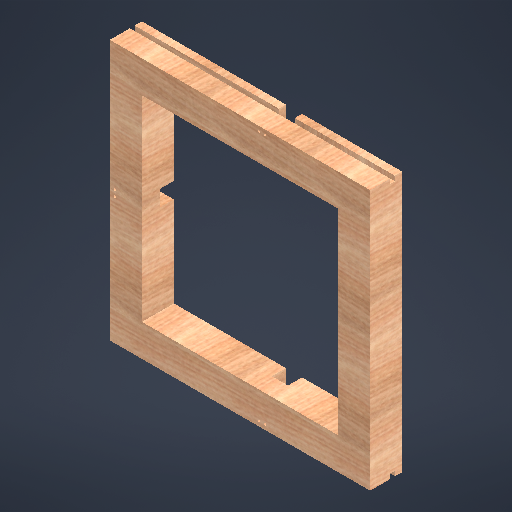
# Autodesk Inventor part: Rahmen_Unten
Saved by Autodesk Inventor 2026.2 (Build 302298000, 298)
## iProperties
Created: 2026-01-27
Part Number: Rahmen_Unten
Material: Holz (Birke)
Document SubType Name: Modeling
Designer: Alex
Density: 0.55 g/cm^3
Appearance: Birke - natur - poliert
Author: Alex
Autodesk Inventor part; units mm, degrees
ref_plane "YZ Plane" through (0, 0, 0) normal (1, 0, 0) x (0, 1, 0)
ref_plane "XZ Plane" through (0, 0, 0) normal (0, 1, 0) x (-1, 0, 0)
ref_plane "XY Plane" through (0, 0, 0) normal (0, 0, 1) x (1, 0, 0)
sketch "Skizze1" plane through (0, 0, 0) normal (0, 1, 0) x (-1, 0, 0)
  line L0 (0, 0) -> (80, 0)
  line L1 (80, 0) -> (80, -650)
  line L2 (80, -650) -> (0, -650)
  line L3 (0, -650) -> (0, 0)
  line L4 (80, -570) -> (80, -650)
  line L5 (80, -650) -> (570, -650)
  line L6 (570, -650) -> (570, -570)
  line L7 (570, -570) -> (80, -570)
  line L8 (80, -570) -> (80, -650)
  line L9 (80, 0) -> (570, 0)
  line L10 (570, 0) -> (570, -80)
  line L11 (570, -80) -> (80, -80)
  line L12 (80, -80) -> (80, 0)
  line L13 (570, 0) -> (650, 0)
  line L14 (650, 0) -> (650, -650)
  line L15 (650, -650) -> (570, -650)
  line L16 (570, -650) -> (570, 0)
  dimension "d0" = 80
  dimension "d1" = 650
  dimension "d4" = 490
  dimension "d5" = 80
  dimension "d6" = 80
  dimension "d7" = 80
  constraints: 34 end point, 8 parallel, 4 horizontal, 4 perpendicular, 2 point on line
  measures "d0" distance of L1.end L2.end
  measures "d1" distance of L0.end L1.end
  measures "d4" distance of L7.end L6.end
  measures "d5" distance of L6.end L5.end
  measures "d6" distance of L9.end L10.end
  measures "d7" distance of L14.end L15.end
extrude "Extrusion1" add sketch "Skizze1" along normal blind 80 contours L0 L1 L2 L3 | L9 L10 L11 L1 | L13 L14 L15 L6 L16 L10 | L1 L7 L6 L5
sketch "Skizze2" plane through (0, 80, 0) normal (0, 1, 0) x (1, 0, 0)
  line L0 (0, 0) -> (0, 650) projected
  line L1 (0, 650) -> (-650, 650) projected
  line L2 (-650, 650) -> (-650, 0) projected
  line L3 (-650, 0) -> (0, 0) projected
  line L4 (-80, 80) -> (-570, 80) projected
  line L5 (-570, 80) -> (-570, 570) projected
  line L6 (-570, 570) -> (-80, 570) projected
  line L7 (-80, 570) -> (-80, 80) projected
  line L8 (-490, 305) -> (-490, 345)
  line L9 (-490, 345) -> (-650, 345)
  line L10 (-650, 345) -> (-650, 305)
  line L11 (-650, 305) -> (-490, 305)
  line L12 (-570, 80) -> (-570, 570) projected
  line L13 (-490, 305) -> (-650, 345) construction
  line L14 (-490, 345) -> (-650, 305) construction
  line L15 (-80, 80) -> (-570, 80) projected
  line L16 (-570, 80) -> (-270, 80)
  line L17 (-250, 160) -> (-290, 160)
  line L18 (-290, 160) -> (-290, 0)
  line L19 (-290, 0) -> (-250, 0)
  line L20 (-250, 0) -> (-250, 160)
  line L21 (-250, 160) -> (-290, 0) construction
  line L22 (-290, 160) -> (-250, 0) construction
  line L23 (-650, 325) -> (0, 325)
  line L24 (-250, 490) -> (-290, 490)
  line L25 (-290, 490) -> (-290, 650)
  line L26 (-250, 650) -> (-250, 490)
  line L27 (-290, 650) -> (-250, 650)
  point P0 (-570, 325)
  point P1 (-250, 570)
  point P2 (-290, 570)
  point P3 (-570, 345)
  point P4 (-570, 305)
  point P5 (-250, 80)
  point P6 (-290, 80)
  dimension "d10" = 40
  dimension "d11" = 300
  dimension "d12" = 40
  constraints: 36 end point, 7 midpoint, 4 parallel, 4 symmetric about line, 2 perpendicular, 1 collinear, 1 point on line
  measures "d10" distance of L8.start L8.end
  measures "d11" distance of L4.end L16.end
  measures "d12" distance of L17.start L17.end
extrude "Extrusion2" cut sketch "Skizze2" against normal blind 30 contours L3 L18 L4 L20 | L26 L6 L25 L1 | L23 L2 L9 L5 | L5 L11 L2 L23
sketch "Skizze3" plane through (0, 50, 0) normal (0, 1, 0) x (1, 0, 0)
  line L0 (-290, 80) -> (-250, 80) projected
  line L1 (-290, 0) -> (-290, 80) projected
  line L2 (-250, 0) -> (-290, 0) projected
  line L3 (-250, 80) -> (-250, 0) projected
  line L4 (-290, 650) -> (-250, 650) projected
  line L5 (-290, 570) -> (-290, 650) projected
  line L6 (-250, 570) -> (-290, 570) projected
  line L7 (-250, 650) -> (-250, 570) projected
  line L8 (-650, 345) -> (-570, 345) projected
  line L9 (-650, 305) -> (-650, 345) projected
  line L10 (-570, 305) -> (-650, 305) projected
  line L11 (-570, 345) -> (-570, 305) projected
  line L12 (-650, 305) -> (-625, 305)
  line L13 (-570, 305) -> (-650, 305) projected
  line L14 (-625, 305) -> (-625, 345)
  line L15 (-290, 650) -> (-290, 625)
  line L16 (-290, 570) -> (-290, 650) projected
  line L17 (-290, 625) -> (-250, 625)
  line L18 (-290, 0) -> (-290, 25)
  line L19 (-290, 25) -> (-250, 25)
  point P0 (0, 0)
  dimension "d15" = 25
  dimension "d16" = 25
  dimension "d17" = 25
  constraints: 12 end point, 6 point on line, 3 perpendicular
  measures "d15" distance of L9.start L12.end
  measures "d16" distance of L4.start L15.end
  measures "d17" distance of L1.start L18.end
extrude "Extrusion3" cut sketch "Skizze3" against normal blind 5 contours L0 L3 L19 L1 | L17 L7 L6 L5 | L8 L11 L10 L14
sketch "Skizze4" plane through (0, 0, -650) normal (0, 0, -1) x (-1, 0, 0)
  line L0 (290, 80) -> (290, 50) projected
  line L1 (290, 50) -> (250, 50) projected
  line L2 (250, 50) -> (250, 80) projected
  line L3 (0, 80) -> (250, 80) projected
  line L4 (0, 0) -> (0, 80) projected
  line L5 (0, 0) -> (650, 0) projected
  line L6 (650, 0) -> (650, 80) projected
  line L7 (290, 80) -> (650, 80) projected
  line L8 (250, 50) -> (250, 45) projected
  line L9 (250, 50) -> (0, 50)
  line L10 (0, 0) -> (0, 80) projected
  line L11 (290, 50) -> (250, 50) projected
  line L12 (250, 50) -> (250, 62)
  line L13 (250, 62) -> (0, 62)
  line L14 (290, 50) -> (650, 50)
  line L15 (290, 62) -> (650, 62)
  dimension "d20" = 12
  constraints: 10 end point, 7 point on line, 3 perpendicular
  measures "d20" distance of L1.end L12.end
extrude "Extrusion4" cut sketch "Skizze4" against normal blind 12 contours L15 L6 L14 L0 | L9 L4 L13 L2
sketch "Skizze5" plane through (-650, 0, -650) normal (-1, 0, 0) x (0, 0, 1)
  line L0 (12, 50) -> (0, 50) projected
  line L1 (0, 0) -> (0, 50) projected
  line L2 (0, 0) -> (650, 0) projected
  line L3 (650, 0) -> (650, 80) projected
  line L4 (345, 80) -> (650, 80) projected
  line L5 (345, 80) -> (345, 50) projected
  line L6 (345, 50) -> (305, 50) projected
  line L7 (305, 50) -> (305, 80) projected
  line L8 (0, 80) -> (305, 80) projected
  line L9 (0, 62) -> (0, 80) projected
  line L10 (0, 62) -> (12, 62) projected
  line L11 (12, 62) -> (12, 50) projected
  line L12 (12, 50) -> (650, 50)
  line L13 (12, 62) -> (650, 62)
  point P0 (345, 62)
  point P1 (305, 62)
  constraints: 4 end point, 2 perpendicular, 2 point on line
extrude "Extrusion5" cut sketch "Skizze5" against normal blind 12 contours L11 L13 L7 L12 | L5 L13 L3 L12
sketch "Skizze6" plane through (-650, 0, 0) normal (0, 0, 1) x (1, 0, 0)
  line L0 (12, 50) -> (12, 62) projected
  line L1 (12, 50) -> (650, 50)
  line L2 (360, 62) -> (12, 62) projected
  line L3 (650, 62) -> (400, 62) projected
  line L4 (12, 50) -> (0, 50) projected
  line L5 (0, 0) -> (0, 50) projected
  line L6 (0, 0) -> (650, 0) projected
  line L7 (650, 0) -> (650, 80) projected
  line L8 (400, 80) -> (650, 80) projected
  line L9 (400, 80) -> (400, 50) projected
  line L10 (400, 50) -> (360, 50) projected
  line L11 (360, 50) -> (360, 80) projected
  line L12 (0, 80) -> (360, 80) projected
  line L13 (0, 62) -> (0, 80) projected
  line L14 (0, 62) -> (12, 62) projected
  line L15 (12, 62) -> (12, 50) projected
  constraints: 2 end point
extrude "Extrusion6" cut sketch "Skizze6" against normal blind 12 contours L0 L2 L11 L1 | L9 L3 L7 L1
sketch "Skizze7" plane through (0, 0, -650) normal (0, 0, -1) x (-1, 0, 0)
  line L0 (650, 50) -> (0, 50) projected
  line L1 (0, 0) -> (0, 50) projected
  line L2 (0, 0) -> (650, 0) projected
  line L3 (650, 0) -> (650, 50) projected
  line L4 (0, 50) -> (0, 62) projected
  line L5 (250, 50) -> (0, 50) projected
  line L6 (250, 62) -> (250, 50) projected
  line L7 (0, 62) -> (250, 62) projected
  line L8 (0, 62) -> (250, 62) projected
  line L9 (250, 62) -> (250, 80) projected
  line L10 (0, 80) -> (250, 80) projected
  line L11 (0, 62) -> (0, 80) projected
  line L12 (290, 62) -> (650, 62) projected
  line L13 (650, 62) -> (650, 80) projected
  line L14 (290, 80) -> (650, 80) projected
  line L15 (290, 80) -> (290, 62) projected
  line L16 (638, 50) -> (638, 62) projected
  line L17 (290, 62) -> (638, 62) projected
  line L18 (290, 50) -> (290, 62) projected
  line L19 (638, 50) -> (290, 50) projected
  line L20 (250, 50) -> (200, 50)
  line L21 (290, 50) -> (340, 50)
  line L22 (250, 50) -> (290, 50) projected
  ellipse E0 centre (270, 50) end of major axis (200, 50) minor radius 17.9197
  line L23 (200, 50) -> (188, 50)
  line L24 (250, 62) -> (0, 62) projected
  line L25 (218.0128, 62) -> (213.5364, 73.1338)
  ellipse E1 centre (270, 50) end of major axis (188, 50) minor radius 28.5733
  point P0 (352, 50)
  dimension "d27" = 50
  dimension "d28" = 50
  dimension "d29" = 12
  dimension "d30" = 12
  constraints: 8 end point, 4 point on line, 2 horizontal, 1 coincident, 1 midpoint, 7 other
  measures "d27" distance of L5.start L20.end
  measures "d28" distance of L18.start L21.end
  measures "d29" distance of L20.end L23.end
  measures "d30" distance of L25.start L25.end
extrude "Extrusion7" cut sketch "Skizze7" against normal blind 12 contours E1 L0 E0
sketch "Skizze8" plane through (0, 50, 0) normal (0, 1, 0) x (1, 0, 0)
  line L0 (-352, 638) -> (-352, 650) projected
  line L1 (-650, 650) -> (-352, 650) projected
  line L2 (-650, 0) -> (-650, 650) projected
  line L3 (0, 0) -> (-650, 0) projected
  line L4 (0, 12) -> (0, 0) projected
  line L5 (0, 12) -> (-250, 12) projected
  line L6 (-250, 25) -> (-250, 12) projected
  line L7 (-250, 25) -> (-290, 25) projected
  line L8 (-290, 12) -> (-290, 25) projected
  line L9 (-290, 12) -> (-638, 12) projected
  line L10 (-638, 12) -> (-638, 305) projected
  line L11 (-625, 305) -> (-638, 305) projected
  line L12 (-625, 305) -> (-625, 345) projected
  line L13 (-638, 345) -> (-625, 345) projected
  line L14 (-638, 345) -> (-638, 638) projected
  line L15 (-638, 638) -> (-352, 638) projected
  line L16 (-290, 25) -> (-290, 80) projected
  line L17 (-250, 25) -> (-290, 25) projected
  line L18 (-250, 80) -> (-250, 25) projected
  line L19 (-290, 80) -> (-250, 80) projected
  line L20 (-290, 0) -> (-290, 12) projected
  line L21 (-290, 12) -> (-290, 0)
  line L22 (0, 12) -> (-250, 12) projected
  line L23 (-250, 80) -> (-250, 0) projected
  line L24 (-250, 12) -> (-250, 0)
  line L25 (-250, 12) -> (-262.5, 12)
  line L26 (-262.5, 12) -> (-277.5, 12)
  circle A0 centre (-277.5, 12) radius 3
  circle A1 centre (-262.5, 12) radius 3
  line L27 (-638, 305) -> (-638, 317.5)
  line L28 (-638, 317.5) -> (-638, 332.5)
  circle A2 centre (-638, 317.5) radius 3
  circle A3 centre (-638, 332.5) radius 3
  line L29 (-340, 650) -> (-340, 638) projected
  line L30 (-340, 638) -> (-290, 638) projected
  line L31 (-290, 625) -> (-290, 638) projected
  line L32 (-290, 625) -> (-250, 625) projected
  line L33 (-250, 638) -> (-250, 625) projected
  line L34 (-250, 638) -> (-200, 638) projected
  line L35 (-200, 638) -> (-200, 650) projected
  line L36 (-340, 650) -> (-200, 650) projected
  line L37 (-290, 638) -> (-290, 625.5)
  line L38 (-290, 570) -> (-290, 650) projected
  line L39 (-290, 638) -> (-277.5, 638)
  line L40 (-277.5, 638) -> (-262.5, 638)
  circle A4 centre (-277.5, 638) radius 3
  circle A5 centre (-262.5, 638) radius 3
  dimension "d35" = 12.5
  dimension "d36" = 15
  dimension "d37" = 6
  dimension "d38" = 6
  dimension "d39" = 12.5
  dimension "d40" = 15
  dimension "d41" = 6
  dimension "d42" = 6
  dimension "d43" = 12.5
  dimension "d44" = 12.5
  dimension "d45" = 15
  dimension "d46" = 6
  dimension "d47" = 6
  constraints: 18 end point, 6 centre point, 6 coincident, 4 point on line, 2 collinear, 2 perpendicular, 1 horizontal
  measures "d35" distance of L5.end L25.end
  measures "d36" distance of L25.end L26.end
  measures "d37" diameter of A0
  measures "d38" diameter of A1
  measures "d39" distance of L10.end L27.end
  measures "d40" distance of L27.end L28.end
  measures "d41" diameter of A2
  measures "d42" diameter of A3
  measures "d43" distance of L30.end L37.end
  measures "d44" distance of L30.end L39.end
  measures "d45" distance of L39.end L40.end
  measures "d46" diameter of A4
  measures "d47" diameter of A5
extrude "Extrusion8" cut sketch "Skizze8" against normal blind 100 contours A3 | A2 L28 L27 | L27 L28 A2 | A0 | A1 L26 L25 | L25 L26 A1 | A5 | A4 L40 L39 | L39 L40 A4
